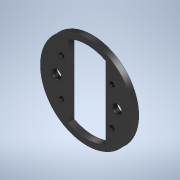
# Autodesk Inventor part: CarriageCap_V4
Saved by Autodesk Inventor 2020 (Build 240168000, 168)
## iProperties
Created: 2020-01-04
Part Number: CarriageCap_V4
Material: ABS Plastic
Document SubType Name: Modeling
Designer: Connor
Density: 1.06 g/cm^3
Appearance: Glossy - Black
Author: Connor
Autodesk Inventor part; units mm, degrees
ref_plane "YZ Plane" through (0, 0, 0) normal (1, 0, 0) x (0, 1, 0)
ref_plane "XZ Plane" through (0, 0, 0) normal (0, 1, 0) x (-1, 0, 0)
ref_plane "XY Plane" through (0, 0, 0) normal (0, 0, 1) x (1, 0, 0)
sketch "Sketch1" plane through (0, 0, 0) normal (0, 1, 0) x (-1, 0, 0)
  line L0 (0, 0) -> (-46.99, 0)
  line L1 (-46.99, 0) -> (-46.99, -5.5563)
  line L2 (-46.99, -5.5563) -> (0, -5.5562)
  line L3 (0, -5.5562) -> (0, 0)
  line L4 (-44.45, -4.1049) -> (-42.2049, -6.35)
  line L5 (-42.2049, -6.35) -> (-44.45, -8.5951)
  line L6 (-44.45, -8.5951) -> (-46.6951, -6.35)
  line L7 (-46.6951, -6.35) -> (-44.45, -4.1049)
  line L8 (-42.2049, -6.35) -> (0, -6.35)
  line L9 (0, -6.35) -> (0, -5.5562)
  point P0 (-44.45, -6.35)
  point P1 (-45.9013, -5.5563)
  dimension "d0" = 46.99
  dimension "d2" = 3.175
  dimension "d3" = 6.35
  dimension "d4" = 44.45
  dimension "d10" = 0.7937
  constraints: 20 end point, 4 perpendicular, 2 horizontal, 1 vertical alignment, 9 other
  measures "d0" distance of L0.start L0.end
  measures "d2" distance between parallel lines of L7 L5
  measures "d3" distance from line of L0 point (-44.45, -6.35)
  measures "d4" distance from line of L3 point (-44.45, -6.35)
  measures "d10" distance between parallel lines of L8 L2
revolve "Revolution1" add sketch "Sketch1" angle 360 about axis through (0, 0, -5.5562) along (0, 0, 1) contours L3 L2 L4 L7 L1 L0 | L9 L8 L4 L2
sketch "Sketch2" plane through (0, 0, 0) normal (0, 0, 1) x (1, 0, 0)
  circle A0 centre (0, 0) radius 41.275
  line L0 (-19.05, 36.6159) -> (-19.05, -36.6159)
  line L1 (19.05, -36.6159) -> (19.05, 36.6159)
  point P0 (0, 0)
  dimension "d6" = 82.55
  dimension "d7" = 38.1
  constraints: 4 end point, 4 point on circle, 2 vertical, 1 centre point, 1 coincident, 1 parallel
  measures "d6" diameter of A0
  measures "d7" distance between parallel lines of L1 L0
extrude "Extrusion1" cut sketch "Sketch2" against normal through all contours L1 A0 L0
sketch "Sketch3" plane through (0, 0, 0) normal (0, 0, 1) x (1, 0, 0)
  line L0 (25.4, -19.05) -> (-25.4, -19.05) construction
  line L1 (-25.4, -19.05) -> (-25.4, 19.05) construction
  line L2 (-25.4, 19.05) -> (25.4, 19.05) construction
  line L3 (25.4, 19.05) -> (25.4, -19.05) construction
  line L4 (25.4, -19.05) -> (-25.4, 19.05) construction
  line L5 (25.4, 19.05) -> (-25.4, -19.05) construction
  point P0 (0, 0)
  point P1 (0, 0)
  dimension "d11" = 50.8
  dimension "d12" = 38.1
  constraints: 12 end point, 2 parallel, 1 coincident, 1 horizontal, 1 midpoint, 1 perpendicular
  measures "d11" distance of L1.end L2.end
  measures "d12" distance of L0.end L1.end
hole "Hole1" at (25.4, -19.05, 0) at (25.4, 19.05, 0) at (-25.4, 19.05, 0) at (-25.4, -19.05, 0) direction (0, 0, -1) diameter 5.207 end through all
sketch "Sketch4" plane through (0, 0, -6.35) normal (0, 0, -1) x (-1, 0, 0)
  circle A0 centre (0, 0) radius 30.48 construction
  point P0 (0, 0)
  point P1 (-30.48, 0)
  point P2 (30.48, 0)
  dimension "d20" = 60.96
  constraints: 2 point on circle, 1 centre point, 1 coincident
  measures "d20" diameter of A0
hole "Hole2" at (30.48, 0, -6.35) at (-30.48, 0, -6.35) direction (0, 0, 1) diameter 9.525 end through all counterbore diameter 12.954 counterbore depth 4.7752
body "Solid1"
